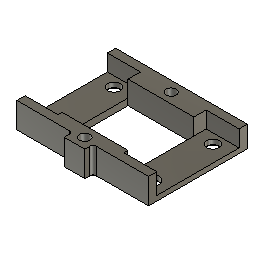
PCB_Stabilizer (Autodesk Fusion 360 design; units mm, degrees)
Autodesk Fusion 360 part; units mm, degrees
note: some values were not read from the file. Set by a fixed rule: which sketch regions a step uses.
sketch "Sketch1" plane through (0, 0, 0) normal (0, 0, 1) x (1, 0, 0)
  line L0 (0, 0) -> (8, 0)
  line L1 (8, 0) -> (8, 24)
  line L2 (8, 24) -> (0, 24)
  line L3 (0, 24) -> (0, 0)
  line L4 (0, 2) -> (8, 2)
  line L5 (0, 22) -> (8, 22)
  line L6 (4, 22) -> (4, 2) construction
  circle A0 centre (4, 4.38) radius 2
  circle A1 centre (4, 19.62) radius 1.525
  line L7 (4, 12) -> (8, 12) construction
  dimension "d1" = 8
  dimension "d2" = 24
  dimension "d3" = 2
  dimension "d4" = 2
  dimension "d5" = 7.62
  dimension "d6" = 7.62
  dimension "d7" = 4
  dimension "d8" = 3.05
  measures "d1" distance of L0.start
  measures "d3" distance of L2 L5
  measures "d4" distance of L0 L4
  measures "d7" diameter of A0
  measures "d8" diameter of A1
extrude "Extrude1" add sketch "Sketch1" along normal blind 1.6 makes body 1
extrude "Extrude2" add sketch "Sketch1" along normal blind 5.6 contours L0 L1 L3 L4 | L1 L2 L3 L5 bodies 1
ref_plane "WorkPlane1" through (-8, 12, 3) normal (-1, 0, 0) x (0, -1, 0)
mirror "Mirror1" about plane through (-8, 12, 3) normal (-1, 0, 0) of bodies 1 makes body 2
sketch "Sketch2" plane through (0, 0, 0) normal (0, 0, -1) x (1, 0, 0)
  line L0 (0, -24) -> (0, 0) construction
  line L1 (-16, -24) -> (-16, 0) construction
  line L2 (-16, 0) -> (0, 0)
  line L3 (0, 0) -> (0, -3)
  line L4 (0, -3) -> (-16, -3)
  line L5 (-16, -3) -> (-16, 0)
  line L6 (-16, -24) -> (0, -24)
  line L7 (0, -24) -> (0, -19)
  line L8 (0, -19) -> (-16, -19)
  line L9 (-16, -19) -> (-16, -24)
  dimension "d16" = 3
  dimension "d17" = 5
extrude "Extrude3" add sketch "Sketch2" against normal up to surface (5.6 mm away) bodies 1 2
sketch "Sketch3" plane through (0, 0, 0) normal (0, 0, -1) x (1, 0, 0)
  line L0 (-24, 0) -> (8, 0) construction
  line L1 (8, -24) -> (-24, -24) construction
  line L2 (-8, 0) -> (-8, -24) construction
  circle A0 centre (-8, -21.5) radius 1.25
  line L3 (-10.5, 2) -> (-5.5, 2)
  line L4 (-5.5, 2) -> (-5.5, 0)
  line L5 (-5.5, 0) -> (-10.5, 0)
  line L6 (-10.5, 0) -> (-10.5, 2)
  circle A1 centre (-8, -0.5) radius 1.25
  dimension "d20" = 2.5
  dimension "d21" = 5
  dimension "d22" = 2
  dimension "d25" = 2.5
  dimension "d26" = 2.5
  dimension "d27" = 2.5
  measures "d20" diameter of A0
  measures "d25" diameter of A1
  measures "d26" distance of L3
  measures "d27" distance of L1
extrude "Extrude4" add sketch "Sketch3" against normal up to surface (5.6 mm away) contours L3 L4 L5 L6 A1 | L5 A1 picked at (-7.7238, 0.1453) bodies 1
extrude "Extrude5" cut sketch "Sketch3" against normal blind 11 contours A0 | L5 A1 | L5 A1 bodies 1
sketch "Sketch5" plane through (0, 0, 0) normal (0, 0, -1) x (1, 0, 0)
  circle A0 centre (-8, -0.5) radius 1.25 construction
  circle A1 centre (-8, -21.5) radius 1.25 construction
  circle A2 centre (-8, -21.5) radius 2
  circle A3 centre (-8, -0.5) radius 2
  dimension "d38" = 4
  dimension "d39" = 4
  measures "d38" diameter of A2
  measures "d39" diameter of A3
extrude "Extrude7" cut sketch "Sketch5" against normal blind 2 bodies 1
fillet "Fillet2" radius 0.8 2 edges at (-5.5, 0, 2.8) (-10.5, 0, 2.8) on bodies 1
chamfer "Chamfer2" distance 0.4 angle 45 14 edges at (-17.65, 0, 0) (-10.7343, -0.2343, 0) (-10.5, -1.4, 0) (-8, -2, 0) (-5.5, -1.4, 0) (-5.2657, -0.2343, 0) (1.65, 0, 0) (-24, 12, 0) (-8, 24, 0) (8, 12, 0) (2.5782, 20.1715, 0) (2.1353, 5.1032, 0) (-18.1353, 5.1032, 0) (-18.5782, 20.1715, 0) on bodies 1
extrude "Extrude8" add 1 faces at (-17.1, 0.6667, 5.6) along direction (0, 0, 1) blind 1 on bodies 1 bodies 1
extrude "Extrude9" cut 1 faces at (-6.2621, 0.6615, 2) along direction (0, 0, 1) blind 1 on bodies 1 bodies 1
chamfer "Chamfer6" distance 0.75 angle 45 2 edges at (-9.1654, 0.952, 3) (-9.1654, 21.952, 2) on bodies 1
equation "d11 = 1.6 mm + 4 mm"
named bodies: "StabAdaptor", "StabAdaptor (1)"
